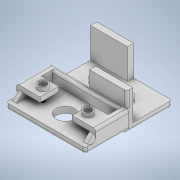
# Autodesk Inventor part: T-RodBot
Saved by Autodesk Inventor 2022 (Build 260153000, 153)
## iProperties
Created: 2020-10-30
Part Number: T-RodBot
Material: Generic
Document SubType Name: Modeling
Designer: PAB
Density: 1 g/cm^3
Appearance: Default
Author: PAB
Autodesk Inventor part; units mm, degrees
ref_plane "YZ Plane" through (0, 0, 0) normal (1, 0, 0) x (0, 1, 0)
ref_plane "XZ Plane" through (0, 0, 0) normal (0, 1, 0) x (-1, 0, 0)
ref_plane "XY Plane" through (0, 0, 0) normal (0, 0, 1) x (1, 0, 0)
sketch "Sketch1" plane through (0, 0, 0) normal (0, 1, 0) x (-1, 0, 0)
  line L0 (30.4, 18.2) -> (-30.4, 18.2)
  line L1 (-30.4, 18.2) -> (-30.4, -18.2)
  line L2 (-30.4, -18.2) -> (30.4, -18.2)
  line L3 (30.4, -18.2) -> (30.4, 18.2)
  point P0 (0, 0)
  dimension "d0" = 60.8
  dimension "d1" = 36.4
  constraints: 8 end point, 2 parallel, 1 horizontal, 1 perpendicular
  measures "d0" distance of L2.end L1.end
  measures "d1" distance of L1.end L0.end
extrude "Extrusion1" add sketch "Sketch1" along normal blind 5
sketch "Sketch2" plane through (0, 5, 0) normal (0, 1, 0) x (1, 0, 0)
  line L0 (30.4, 18.2) -> (-30.4, 18.2) projected
  line L1 (-30.4, 18.2) -> (-0.4, 18.2)
  line L2 (-0.4, 18.2) -> (-0.4, 13.2)
  line L3 (-0.4, 13.2) -> (-30.4, 13.2)
  line L4 (-30.4, 13.2) -> (-30.4, 18.2)
  line L5 (30.4, -18.2) -> (30.4, 18.2) projected
  line L6 (30.4, -18.2) -> (0.4, -18.2)
  line L7 (0.4, -18.2) -> (0.4, -13.2)
  line L8 (0.4, -13.2) -> (30.4, -13.2)
  line L9 (30.4, -13.2) -> (30.4, -18.2)
  point P0 (0, 0)
  dimension "d4" = 30
  dimension "d5" = 5
  dimension "d6" = 30
  dimension "d7" = 5
  constraints: 16 end point, 4 parallel, 2 horizontal, 2 perpendicular
  measures "d4" distance of L2.end L3.end
  measures "d5" distance of L1.end L2.end
  measures "d6" distance of L7.end L8.end
  measures "d7" distance of L6.end L7.end
extrude "Extrusion2" add sketch "Sketch2" along normal blind 24.4
sketch "Sketch3" plane through (0, 5, 0) normal (0, 1, 0) x (1, 0, 0)
  circle A0 centre (12.7, 0) radius 4.325
  circle A1 centre (-12.7, 0) radius 4.325
  point P0 (0, 0)
  dimension "d10" = 8.65
  dimension "d11" = 8.65
  constraints: 2 centre point
  measures "d10" diameter of A0
  measures "d11" diameter of A1
extrude "Extrusion3" add sketch "Sketch3" along normal blind 5
sketch "Sketch4" plane through (-12.7, 10, 0) normal (0, 1, 0) x (1, 0, 0)
  circle A0 centre (0, 0) radius 2
  circle A1 centre (25.4, 0) radius 4.325 projected
  circle A2 centre (25.4, 0) radius 2
  point P0 (12.7, 0)
  dimension "d14" = 4
  dimension "d15" = 4
  constraints: 2 centre point, 1 coincident
  measures "d14" diameter of A0
  measures "d15" diameter of A2
extrude "Extrusion4" cut sketch "Sketch4" against normal blind 15 contours A0 | A2
sketch "Sketch5" plane through (0, 0, 0) normal (0, -1, 0) x (1, 0, 0)
  circle A0 centre (12.7, 0) radius 2 projected
  circle A1 centre (12.7, 0) radius 3
  circle A2 centre (-12.7, 0) radius 2 projected
  circle A3 centre (-12.7, 0) radius 3
  point P0 (0, 0)
  dimension "d18" = 6
  dimension "d19" = 6
  constraints: 2 centre point, 2 coincident
  measures "d18" diameter of A1
  measures "d19" diameter of A3
extrude "Extrusion5" cut sketch "Sketch5" against normal blind 3 contours A0 | A1 | A2 | A3
chamfer "Chamfer1" distance 1.5 angle 45 2 edges at (8.375, 10, 0) (-17.025, 10, 0)
sketch "Sketch6" plane through (-30.4, 0, 18.2) normal (0, 0, 1) x (1, 0, 0)
  line L0 (-1.6, 3) -> (62.4, 3)
  line L1 (62.4, 3) -> (62.4, 8)
  line L2 (62.4, 8) -> (-1.6, 8)
  line L3 (-1.6, 8) -> (-1.6, 3)
  point P0 (30.4, 0)
  dimension "d26" = 64
  dimension "d27" = 5
  constraints: 8 end point, 2 parallel, 1 horizontal, 1 perpendicular
  measures "d26" distance of L2.end L1.end
  measures "d27" distance of L1.end L0.end
extrude "Extrusion6" add sketch "Sketch6" along normal blind 35
chamfer "Chamfer2" distance 3 angle 45 1 edges at (0, 3, 18.2)
sketch "Sketch7" plane through (-32, 8, 18.2) normal (0, 1, 0) x (1, 0, 0)
  line L0 (0, 0) -> (1.6, 0) projected
  line L1 (0, 0) -> (5, 0)
  line L2 (5, 0) -> (5, -26.65)
  line L3 (5, -26.65) -> (0, -26.65)
  line L4 (0, -26.65) -> (0, 0)
  line L5 (64, 0) -> (64, -35) projected
  line L6 (64, 0) -> (59, 0)
  line L7 (59, 0) -> (59, -26.65)
  line L8 (59, -26.65) -> (64, -26.65)
  line L9 (64, -26.65) -> (64, 0)
  line L10 (5, 0) -> (59, 0)
  line L11 (59, 0) -> (59, -3)
  line L12 (59, -3) -> (5, -3)
  line L13 (5, -3) -> (5, 0)
  point P0 (32, 18.2)
  dimension "d33" = 5
  dimension "d34" = 26.65
  dimension "d35" = 5
  dimension "d36" = 3
  constraints: 24 end point, 6 parallel, 3 horizontal, 3 perpendicular, 2 point on line
  measures "d33" distance of L2.end L3.end
  measures "d34" distance of L1.end L2.end
  measures "d35" distance of L8.end L7.end
  measures "d36" distance of L10.end L11.end
extrude "Extrusion7" add sketch "Sketch7" along normal blind 9
sketch "Sketch8" plane through (27, 8, 21.2) normal (-1, 0, 0) x (0, 0, 1)
  line L0 (23.65, 0) -> (23.65, 9) projected
  line L1 (23.65, 9) -> (8.65, 9)
  line L2 (8.65, 9) -> (8.65, 5)
  line L3 (8.65, 5) -> (23.65, 5)
  line L4 (23.65, 5) -> (23.65, 9)
  point P0 (-21.2, -8)
  point P1 (23.65, 5)
  dimension "d39" = 15
  dimension "d40" = 4
  constraints: 8 end point, 2 parallel, 1 horizontal, 1 perpendicular
  measures "d39" distance of L3.end L2.end
  measures "d40" distance of L2.end L1.end
extrude "Extrusion8" add sketch "Sketch8" along normal blind 14
mirror "Mirror1" about plane through (0, 0, 0) normal (1, 0, 0) of "Extrusion8"
sketch "Sketch9" plane through (-32, 17, 18.2) normal (0, 1, 0) x (1, 0, 0)
  circle A0 centre (13.75, -19.15) radius 4
  circle A1 centre (50.25, -19.15) radius 4
  point P0 (32, 18.2)
  dimension "d43" = 8
  dimension "d44" = 8
  constraints: 2 centre point
  measures "d43" diameter of A0
  measures "d44" diameter of A1
extrude "Extrusion9" add sketch "Sketch9" along normal blind 3
sketch "Sketch10" plane through (-32, 8, 53.2) normal (0, 1, 0) x (1, 0, 0)
  circle A0 centre (32, 15.85) radius 7.5
  circle A1 centre (13.75, 15.85) radius 4 projected
  circle A2 centre (13.75, 15.85) radius 2
  circle A3 centre (50.25, 15.85) radius 4 projected
  circle A4 centre (50.25, 15.85) radius 2
  point P0 (32, 53.2)
  dimension "d47" = 15
  dimension "d48" = 4
  dimension "d49" = 4
  constraints: 3 centre point, 2 coincident
  measures "d47" diameter of A0
  measures "d48" diameter of A2
  measures "d49" diameter of A4
extrude "Extrusion10" cut sketch "Sketch10" along normal mid plane 50 contours A0 | A2 | A4
sketch "Sketch11" plane through (-18.25, 20, 37.35) normal (0, 1, 0) x (1, 0, 0)
  circle A0 centre (0, 0) radius 2 projected
  circle A1 centre (0, 0) radius 3
  circle A2 centre (36.5, 0) radius 2 projected
  circle A3 centre (36.5, 0) radius 3
  point P0 (18.25, 37.35)
  dimension "d52" = 6
  dimension "d53" = 6
  constraints: 2 centre point, 2 coincident
  measures "d52" diameter of A1
  measures "d53" diameter of A3
extrude "Extrusion11" cut sketch "Sketch11" against normal blind 3 contours A0 | A1 | A3
chamfer "Chamfer3" distance 5 angle 45 2 edges at (-29.5, 8, 44.85) (29.5, 8, 44.85)
fillet "Fillet2" radius 2 18 edges at (-30.4, 0, 18.2) (-30.4, 0, 0) (0, 0, -18.2) (30.4, 0.0001, 18.2) (30.4, 0, 0) (-30.4, 14.7, -18.2) (30.4, 2.5, -18.2) (30.4, 23.2, 18.2) (-32, 17, 31.525) (32, 17, 31.525) (0, 17, 21.2) (-32, 10.5, 47.35) (32, 10.5, 47.35) (0, 3, 53.2) (-32, 3, 35.7) (32, 3, 35.7) (-32, 5.5, 53.2) (32, 5.5, 53.2)
body "Solid1"
